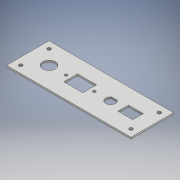
# Autodesk Inventor part: Delta Power Panel ex
Saved by Autodesk Inventor 2018 (Build 220112000, 112)
## iProperties
Created: 2018-04-05
Part Number: Delta Power Panel ex
Material: Generic
Document SubType Name: Modeling
Designer: elect
Density: 1 g/cm^3
Appearance: Default
Author: elect
Autodesk Inventor part; units mm, degrees
ref_plane "YZ Plane" through (0, 0, 0) normal (1, 0, 0) x (0, 1, 0)
ref_plane "XZ Plane" through (0, 0, 0) normal (0, 1, 0) x (-1, 0, 0)
ref_plane "XY Plane" through (0, 0, 0) normal (0, 0, 1) x (1, 0, 0)
sketch "Sketch1" plane through (0, 0, 0) normal (0, 0, 1) x (1, 0, 0)
  line L0 (0, 0) -> (-176, 0)
  line L1 (-176, 0) -> (-176, 60)
  line L2 (-176, 60) -> (0, 60)
  line L3 (0, 60) -> (0, 0)
  line L4 (0, 0) -> (-20, 0)
  line L5 (-20, 0) -> (-20, 30)
  line L6 (-20, 30) -> (0, 30)
  line L7 (0, 30) -> (0, 0)
  line L8 (-176, 0) -> (-156, 0)
  line L9 (-156, 0) -> (-156, 30)
  line L10 (-156, 30) -> (-176, 30)
  line L11 (-176, 30) -> (-176, 0)
  line L12 (-20, 22.5) -> (-41, 22.5)
  line L13 (-41, 22.5) -> (-41, 37.5)
  line L14 (-41, 37.5) -> (-20, 37.5)
  line L15 (-20, 37.5) -> (-20, 22.5)
  line L16 (-20, 22.5) -> (-41, 37.5) construction
  line L17 (-41, 22.5) -> (-20, 37.5) construction
  line L18 (-20, 30) -> (-51, 30)
  line L19 (-51, 30) -> (-66.9, 30)
  line L20 (-66.9, 30) -> (-76.9, 30)
  line L21 (-126.9, 20.25) -> (-76.9, 20.25)
  line L22 (-76.9, 20.25) -> (-76.9, 39.75)
  line L23 (-76.9, 39.75) -> (-126.9, 39.75)
  line L24 (-126.9, 39.75) -> (-126.9, 20.25)
  line L25 (-126.9, 20.25) -> (-76.9, 39.75) construction
  line L26 (-76.9, 20.25) -> (-126.9, 39.75) construction
  line L27 (-76.9, 39.75) -> (-88.4, 39.75)
  line L28 (-88.4, 39.75) -> (-88.4, 20.25)
  line L29 (-88.4, 20.25) -> (-76.9, 20.25)
  line L30 (-76.9, 20.25) -> (-76.9, 39.75)
  line L31 (-88.4, 39.75) -> (-115.4, 39.75)
  line L32 (-115.4, 39.75) -> (-115.4, 20.25)
  line L33 (-115.4, 20.25) -> (-88.4, 20.25)
  line L34 (-88.4, 20.25) -> (-88.4, 39.75)
  line L35 (-101.9, 30) -> (-81.9, 30)
  line L36 (-101.9, 30) -> (-121.9, 30)
  circle A0 centre (-121.9, 30) radius 2
  circle A1 centre (-81.9, 30) radius 2
  line L37 (-126.9, 30) -> (-136.9, 30)
  circle A2 centre (-145.9, 30) radius 9
  circle A3 centre (-145.9, 30) radius 7.5
  arc A4 (-62.9649, 35.5) -> (-54.9351, 35.5) centre (-58.95, 30) ccw
  line L38 (-66.9, 60) -> (-51, 60)
  line L39 (-51, 30) -> (-66.9, 30)
  line L40 (-66.9, 60) -> (-51, 60)
  line L41 (-54.9351, 35.5) -> (-62.9649, 35.5)
  circle A5 centre (-10, 10) radius 2.5
  circle A6 centre (-10, 50) radius 2.5
  circle A7 centre (-166, 50) radius 2.5
  circle A8 centre (-166, 10) radius 2.5
  point P0 (-30.5, 30)
  dimension "d0" = 176
  dimension "d1" = 60
  dimension "d2" = 20
  dimension "d3" = 20
  dimension "d4" = 21
  dimension "d5" = 15
  dimension "d6" = 31
  dimension "d8" = 10
  dimension "d9" = 19.5
  dimension "d10" = 11.5
  dimension "d11" = 27
  dimension "d12" = 20
  dimension "d13" = 20
  dimension "d14" = 4
  dimension "d15" = 4
  dimension "d16" = 10
  dimension "d17" = 18
  dimension "d18" = 15
  dimension "d19" = 13.619
  dimension "d21" = 5
  dimension "d22" = 5
  dimension "d23" = 5
  dimension "d24" = 5
  constraints: 84 end point, 16 parallel, 13 horizontal, 9 centre point, 7 perpendicular, 5 midpoint, 5 point on line, 3 coincident, 2 point on circle
  measures "d0" distance of L1.end L2.end
  measures "d1" distance of L0.end L1.end
  measures "d2" distance of L5.end L6.end
  measures "d3" distance of L10.end L9.end
  measures "d4" distance of L13.end L14.end
  measures "d5" distance of L12.end L13.end
  measures "d6" distance of L18.end L5.end
  measures "d8" distance of L19.end L20.end
  measures "d9" distance of L22.end L21.end
  measures "d10" distance of L29.end L28.end
  measures "d11" distance of L33.end L32.end
  measures "d12" distance of L35.start L35.end
  measures "d13" distance of L35.start L36.end
  measures "d14" diameter of A0
  measures "d15" diameter of A1
  measures "d16" distance of L37.start L37.end
  measures "d17" diameter of A2
  measures "d18" diameter of A3
  measures "d19" diameter of A4
  measures "d21" diameter of A5
  measures "d22" diameter of A6
  measures "d23" diameter of A7
  measures "d24" diameter of A8
extrude "Extrusion1" add sketch "Sketch1" along normal blind 2.5 contours L0 L5 L6 L3 | L22 L21 L28 L23 | L0 L9 L10 L1 L2 L3 L6 L15 L14 L13 L12 L5 | L0 L1 L10 L9 | L21 L24 L23 L32
body "Solid1"
